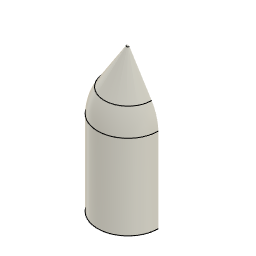
Razzetto 2 v2 (Autodesk Fusion 360 design; units mm, degrees)
Autodesk Fusion 360 part; units mm, degrees
sketch "Schizzo2" plane through (0, 0, 0) normal (0, 1, 0) x (1, 0, 0)
  line L0 (6.25, 0) -> (6.25, -17.4188)
  line L1 (0.2968, -29.5251) -> (4.882, -22.1888)
  line L2 (0, -26.2264) -> (0, -29.6896)
  arc A0 (4.882, -22.1888) -> (6.25, -17.4188) centre (-2.75, -17.4188) ccw
  line L3 (0.9375, -28.5) -> (0, -28.5) construction
  arc A1 (0, -29.6896) -> (0.2968, -29.5251) centre (0, -29.3396) ccw
  line L4 (0, -26.2264) -> (3.186, -21.1288)
  arc A2 (3.186, -21.1288) -> (4.25, -17.4188) centre (-2.75, -17.4188) ccw
  line L5 (4.25, -11.9945) -> (4.25, -17.4188)
  line L6 (4.25, 0) -> (6.25, 0)
  line L7 (4.25, 0) -> (12.7777, 0) construction
  circle A3 centre (0, 0) radius 0.75 construction
  line L8 (4.25, 0) -> (0.75, 0) construction
  line L9 (0.75, 0) -> (0.75, -2.9368) construction
  line L10 (4.25, 0) -> (1.3378, -2.4436)
  line L11 (4.25, 0) -> (9.5183, 0) construction
  line L12 (1.0743, -3.6323) -> (3.5942, -9.0362)
  line L13 (0.75, -2.9368) -> (10.7137, -2.9368) construction
  arc A4 (1.3378, -2.4436) -> (1.0743, -3.6323) centre (1.9806, -3.2097) ccw
  arc A5 (4.25, -11.9945) -> (3.5942, -9.0362) centre (-2.75, -11.9945) ccw
  dimension "d9" = 6.25
  dimension "d15" = 2
  dimension "d24" = 9
  dimension "d25" = 0.35
  dimension "d36" = 1.5
  dimension "d37" = 140
  dimension "d38" = 65
  dimension "d39" = 1
  dimension "d40" = 7
  constraint tangent L1 A0
  constraint tangent L0 A0
  constraint horizontal L3
  constraint coincident L1 L3.start
  constraint coincident L2 L3.end
  constraint tangent L1 A1
  constraint concentric A0 A2
  constraint tangent L4 A2
  constraint tangent A2 L5
  constraint perpendicular L0 L6
  constraint horizontal L7
  constraint coincident A3.centre origin
  constraint coincident A3 L8.end
  constraint tangent A3 L9
  constraint perpendicular L8 L9
  constraint horizontal L11
  constraint horizontal L13
  constraint coincident L10 L9.end
  constraint coincident L9.end L12
  constraint tangent L10 A4
  constraint tangent L12 A4
  constraint tangent L12 A5
  constraint tangent L5 A5
  measures "d9" distance of A3.centre L0.start
  measures "d15" distance of L0.start L6.start
  measures "d24" radius of A0
  measures "d25" radius of A1
  measures "d36" diameter of A3
  measures "d37" angle of L10 L11
  measures "d38" angle of L12 L13
  measures "d39" radius of A4
  measures "d40" radius of A5
revolve "Rivoluzione6" add sketch "Schizzo2" angle 360 about axis through (0, 0, 26.2264) along (0, 0, 1)
revolve "Rivoluzione5" [rolled back] along angle 360
revolve "Rivoluzione3" [suppressed]
ref_plane "Piano di lavoro1" through (0, -3, 0) normal (0, 1, 0) x (0, 0, 1)
revolve "Rivoluzione4" [suppressed]
revolve "Rivoluzione2" [suppressed]
sketch "Schizzo3" plane through (0, 0, 0) normal (0, 1, 0) x (1, 0, 0)
  line L0 (0, 1) -> (0, -23)
  constraint vertical L0
revolve "Rivoluzione1" [suppressed]
equation "d9 = ( 12.5 / 2 ) * 1 mm"
equation "d37 = 180 deg - 40 deg"
named bodies: "razzo", "fiammifero"
